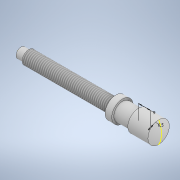
# Autodesk Inventor part: Parafuso2
Saved by Autodesk Inventor 2021 (Build 250183000, 183)
## iProperties
Created: 2022-02-15
Part Number: Parafuso2
Material: Genérico
Document SubType Name: Modeling
Designer: aluno
Density: 1 g/cm^3
Appearance: Padrão
Author: aluno
Autodesk Inventor part; units mm, degrees
ref_plane "YZ Plane" through (0, 0, 0) normal (1, 0, 0) x (0, 1, 0)
ref_plane "XZ Plane" through (0, 0, 0) normal (0, 1, 0) x (-1, 0, 0)
ref_plane "XY Plane" through (0, 0, 0) normal (0, 0, 1) x (1, 0, 0)
sketch "Esboço1" plane through (0, 0, 0) normal (0, 0, 1) x (1, 0, 0)
  line L0 (0, 0) -> (107, 0)
  line L1 (0, 0) -> (2.2532, 3.75)
  line L2 (0, 0) -> (4.3749, 0) construction
  line L3 (2.2532, 3.75) -> (8, 3.75)
  line L4 (8, 3.75) -> (8, 5)
  line L5 (8, 5) -> (73, 5)
  line L6 (73, 5) -> (73, 8)
  line L7 (73, 8) -> (78, 8)
  line L8 (78, 8) -> (78, 6.5)
  line L9 (78, 6.5) -> (90, 6.5)
  line L10 (90, 6.5) -> (90, 8)
  line L11 (90, 8) -> (105, 8)
  arc A0 (107, 0) -> (105, 8) centre (90, 0) ccw
  dimension "d14" = 107
  dimension "d15" = 59
  dimension "d17" = 1.25
  dimension "d18" = 65
  dimension "d19" = 3
  dimension "d20" = 5
  dimension "d21" = 12
  dimension "d22" = 15
  dimension "d24" = 8
  dimension "d25" = 1.5
  dimension "d26" = 7.5
  constraints: 24 end point, 6 perpendicular, 3 horizontal, 3 point on line, 2 point on circle, 1 centre point, 1 equal length, 1 vertical
  measures "d14" distance of L0.start L0.end
  measures "d15" angle of L2 L1
  measures "d17" distance of L3.end L4.end
  measures "d18" distance of L4.end L5.end
  measures "d19" distance of L5.end L6.end
  measures "d20" distance of L6.end L7.end
  measures "d21" distance of L8.end L9.end
  measures "d22" distance of L10.end L11.end
  measures "d24" distance from line of L0.start L4
  measures "d25" distance between parallel lines of L7 L9
  measures "d26" diameter of L3 L0
revolve "Revolução1" add sketch "Esboço1" angle 360 about axis through (0, 0, 0) along (1, 0, 0)
thread "Rosca1" size "M10x1.5" class "6g" standard "ANSI Metric M Profile" full length
sketch "Esboço3" plane through (0, 0, 0) normal (0, 0, 1) x (1, 0, 0)
  circle A0 centre (99, 0) radius 3.25
  arc A1 (105, -8) -> (105, 8) centre (90, 0) ccw projected
  arc A2 (105, -8) -> (105, 8) centre (90, 0) ccw projected
  line L0 (105, -8) -> (105, 8) projected
  point P0 (0, 0)
  dimension "d30" = 6.5
  dimension "d33" = 9
  constraints: 1 centre point, 1 horizontal alignment
  measures "d30" diameter of A0
  measures "d33" distance of A1.centre A0.centre
